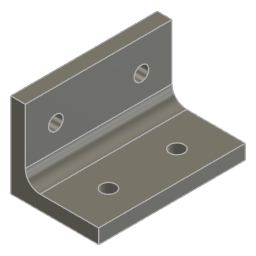
soporte motores (Autodesk Fusion 360 design; units mm, degrees)
part number: 2026-06-22-17-12-05-957
Autodesk Fusion 360 part; units mm, degrees
sketch "Boceto1" plane through (0, 0, 0) normal (0, 0, 1) x (1, 0, 0)
  line L0 (0, 0) -> (3, 0)
  line L1 (3, 0) -> (3, 22.4)
  line L2 (3, 22.4) -> (0, 22.4)
  line L3 (0, 22.4) -> (0, 0)
  dimension "d1" = 3
  dimension "d2" = 22.4
  constraint horizontal L0
  constraint vertical L1
  constraint horizontal L2
  constraint vertical L3
  constraint coincident L0.start L3.end
  measures "d1" distance of L0.start L0.end
  measures "d2" distance of L0.start L2.end
extrude "Extruir1" add sketch "Boceto1" along normal blind 30
sketch "Boceto2" plane through (3, 0, 0) normal (1, 0, 0) x (0, 0, -1)
  line L0 (0, 0) -> (0, 22.4)
  line L1 (0, 22.4) -> (-30, 22.4)
  line L2 (-30, 22.4) -> (-30, 0)
  line L3 (-30, 0) -> (0, 0)
  circle A0 centre (-23.75, 11) radius 1.65
  circle A1 centre (-6.25, 11) radius 1.65
  dimension "d7" = 3.3
  dimension "d8" = 3.3
  measures "d7" diameter of A0
  measures "d8" diameter of A1
hole "Agujero1" at (3, 11, 23.75) at (3, 11, 6.25) direction (-1, 0, 0) diameter 3 depth 10 tip angle 118
sketch "Boceto3" plane through (3, 0, 0) normal (1, 0, 0) x (0, 0, -1)
  circle A0 centre (-23.75, 11) radius 1.5
  circle A1 centre (-6.25, 11) radius 1.5
  line L0 (0, 0) -> (0, 22.4)
  line L1 (0, 22.4) -> (-30, 22.4)
  line L2 (-30, 22.4) -> (-30, 0)
  line L3 (-30, 0) -> (0, 0)
  line L4 (-30, 0) -> (0, 0)
  line L5 (0, 0) -> (0, 3)
  line L6 (0, 3) -> (-30, 3)
  line L7 (-30, 3) -> (-30, 0)
  dimension "d12" = 30
  dimension "d13" = 3
  constraint horizontal L4
  constraint vertical L5
  constraint horizontal L6
  constraint vertical L7
  constraint coincident L2.end L3.start
  measures "d12" distance of L2.end L0.start
  measures "d13" distance of L2.end L6.end
extrude "Extruir2" add sketch "Boceto3" along normal blind 15 contours L0 L2 L3 L4 L5 L6 L7
fillet "Empalme1" radius 3 1 edges at (3, 3, 15)
sketch "Boceto4" plane through (0, 3, 0) normal (0, 1, 0) x (-1, 0, 0)
  line L0 (-6, 0) -> (-6, 30)
  line L1 (-6, 30) -> (-18, 30)
  line L2 (-18, 30) -> (-18, 0)
  line L3 (-18, 0) -> (-6, 0)
  circle A0 centre (-12, 8) radius 1.5
  circle A1 centre (-12, 22) radius 1.5
  dimension "d18" = 3
  dimension "d19" = 3
  measures "d18" diameter of A0
  measures "d19" diameter of A1
hole "Agujero2" at (12, 3, 22) at (12, 3, 8) direction (0, -1, 0) diameter 3 depth 10 tip angle 118
sketch "Boceto5" plane through (3, 0, 0) normal (1, 0, 0) x (0, 0, -1)
  line L0 (-30, 6) -> (0, 6)
  line L1 (0, 6) -> (0, 22.4)
  line L2 (0, 22.4) -> (-30, 22.4)
  line L3 (-30, 22.4) -> (-30, 6)
  circle A0 centre (-23.75, 11) radius 1.5
  circle A1 centre (-6.25, 11) radius 1.5
  line L4 (-30, 22.4) -> (0, 22.4)
  line L5 (0, 22.4) -> (0, 17.4)
  line L6 (0, 17.4) -> (-30, 17.4)
  line L7 (-30, 17.4) -> (-30, 22.4)
  dimension "d23" = 5
  constraint horizontal L4
  constraint vertical L5
  constraint horizontal L6
  constraint vertical L7
  constraint coincident L2.end L3.start
  measures "d23" distance of L2.end L6.end
extrude "Extruir3" cut sketch "Boceto5" against normal blind 9 contours L1 L2 L3 L4 L5 L6 L7
